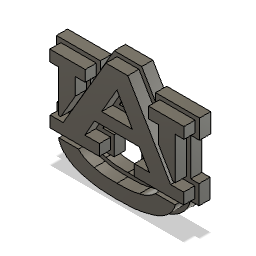
AU_void v3 (Autodesk Fusion 360 design; units mm, degrees)
Autodesk Fusion 360 part; units mm, degrees
sketch "Sketch1" plane through (0, 0, 0) normal (0, 0, 1) x (1, 0, 0)
  line L0 (-1.6004, 6.7897) -> (1.524, 6.7897)
  line L1 (1.524, 6.7897) -> (3.1002, 4.0732)
  line L2 (8.1251, 4.9997) -> (3.1021, 4.9997)
  line L3 (3.1021, 4.9997) -> (3.1002, 4.0732)
  line L4 (8.1251, 4.9997) -> (8.1251, 2.794)
  line L5 (8.1251, 2.794) -> (7.112, 2.794)
  line L6 (7.112, 2.794) -> (7.112, -1.524)
  line L7 (7.112, -1.524) -> (8.0633, -1.524)
  line L8 (8.0633, -1.524) -> (8.0633, -3.7222)
  line L9 (8.0633, -3.7222) -> (7.0698, -3.7222)
  line L10 (3.5709, 4.5364) -> (7.6215, 4.5364)
  line L11 (7.6215, 4.5364) -> (7.6215, 3.2693)
  line L12 (7.6215, 3.2693) -> (6.6294, 3.2693)
  line L13 (6.6294, 3.2693) -> (6.6294, -1.524)
  line L14 (6.6294, -1.524) -> (6.3679, -1.524)
  line L15 (6.3679, -1.524) -> (4.6978, 1.3381)
  line L16 (4.6978, 1.3381) -> (4.6978, 3.2693)
  line L17 (4.6978, 3.2693) -> (3.5709, 3.2693)
  line L18 (3.5709, 3.2693) -> (3.5709, 4.5364)
  line L19 (7.112, 2.794) -> (3.81, 2.794) construction
  line L20 (4.2503, 2.794) -> (4.2503, 2.032) construction
  line L21 (4.0893, 2.3382) -> (3.6031, 3.1299) construction
  line L22 (3.81, 2.794) -> (4.2503, 2.077) construction
  line L23 (4.2503, 2.794) -> (4.2503, 2.077)
  line L24 (3.81, 2.794) -> (4.2503, 2.077)
  line L25 (4.2503, 2.794) -> (4.2503, 2.077)
  line L26 (4.2503, 2.794) -> (3.81, 2.794)
  line L27 (3.81, 2.794) -> (-8.1806, 2.794) construction
  line L28 (-1.7889, 1.3156) -> (1.3724, 6.7897) construction
  line L29 (-1.7889, 1.3156) -> (1.722, 1.3156) construction
  line L30 (-0.0473, 4.3314) -> (1.722, 1.3156) construction
  line L31 (-0.0473, 4.3314) -> (-1.7889, 1.3156)
  line L32 (1.722, 1.3156) -> (-1.7889, 1.3156)
  line L33 (-0.0473, 4.3314) -> (1.722, 1.3156)
  line L34 (-0.0444, 3.4835) -> (0.9772, 1.7422)
  line L35 (-1.05, 1.7422) -> (0.9772, 1.7422)
  line L36 (-1.05, 1.7422) -> (-0.0444, 3.4835)
  line L37 (-0.2083, 6.3583) -> (1.397, 6.3583) construction
  line L38 (6.0908, -1.9713) -> (7.5853, -1.9713) construction
  line L39 (7.5853, -1.9713) -> (7.5853, -3.2478) construction
  line L40 (7.5853, -3.2478) -> (1.9477, -3.2478) construction
  line L41 (1.9477, -3.2478) -> (1.9477, -1.9713) construction
  line L42 (1.9477, -1.9713) -> (6.0908, -1.9713) construction
  line L43 (1.9477, -1.9713) -> (7.5853, -1.9713) construction
  line L44 (7.5853, -1.9713) -> (7.5853, -3.2478) construction
  line L45 (7.5853, -3.2478) -> (1.9477, -3.2478) construction
  line L46 (1.9477, -3.2478) -> (1.9477, -1.9713) construction
  line L47 (1.9477, -1.9713) -> (7.5853, -1.9713)
  line L48 (7.5853, -1.9713) -> (7.5853, -3.2478)
  line L49 (7.5853, -3.2478) -> (1.9477, -3.2478)
  line L50 (1.9477, -3.2478) -> (1.9477, -1.9713)
  line L51 (6.0908, -1.9713) -> (1.1131, 6.5067) construction
  line L52 (-0.0473, 4.3314) -> (-0.0473, 7.112) construction
  line L53 (-0.0473, 6.3583) -> (1.2002, 6.3583)
  line L54 (1.2002, 6.3583) -> (6.0908, -1.9713)
  line L55 (7.0698, -3.7222) -> (1.524, -3.7222) construction
  line L56 (1.524, -3.7222) -> (8.0633, -3.7222)
  line L57 (8.0633, -3.7222) -> (8.0633, -1.524)
  line L58 (8.0633, -1.524) -> (1.524, -1.524)
  line L59 (1.524, -1.524) -> (1.524, -3.7222)
  line L60 (2.8589, -1.524) -> (2.2352, -0.4826)
  line L61 (2.2352, -0.4826) -> (-2.3352, -0.4826) construction
  line L62 (-2.3352, -0.4826) -> (-2.9184, -1.5115) construction
  line L63 (-2.9184, -1.5115) -> (-2.3352, -0.4826)
  line L64 (-2.3352, -0.4826) -> (2.2352, -0.4826)
  line L65 (1.9477, -1.9713) -> (-3.9726, -1.9713) construction
  line L66 (3.2581, -1.2849) -> (2.4989, -0.0173)
  line L67 (-2.6063, -0.0173) -> (2.4989, -0.0173)
  line L68 (-3.717, -1.9768) -> (-2.6063, -0.0173)
  line L69 (-1.6175, -1.9768) -> (-3.717, -1.9768)
  line L70 (-0.0473, 7.112) -> (-0.0473, -8.382)
  line L71 (-0.0473, 6.3583) -> (-1.2948, 6.3583)
  line L72 (-1.2948, 6.3583) -> (-6.1854, -1.9713)
  line L73 (-4.345, 2.794) -> (-3.9046, 2.794)
  line L74 (-3.9046, 2.794) -> (-4.345, 2.077) construction
  line L75 (-4.345, 2.794) -> (-4.345, 2.032) construction
  line L76 (-4.7924, 1.3381) -> (-4.7924, 3.2693)
  line L77 (-4.7924, 3.2693) -> (-3.6655, 3.2693)
  line L78 (-3.6655, 3.2693) -> (-3.6655, 4.5364)
  line L79 (-3.6655, 4.5364) -> (-7.7162, 4.5364)
  line L80 (-7.7162, 4.5364) -> (-7.7162, 3.2693)
  line L81 (-7.7162, 3.2693) -> (-6.724, 3.2693)
  line L82 (-6.724, 3.2693) -> (-6.724, -1.524)
  line L83 (-6.4625, -1.524) -> (-4.7924, 1.3381)
  line L84 (-2.0423, -3.2478) -> (-2.0423, -1.9713)
  line L85 (-7.68, -3.2478) -> (-2.0423, -3.2478)
  line L86 (-2.0423, -1.9713) -> (-7.68, -1.9713)
  line L87 (-7.68, -1.9713) -> (-7.68, -3.2478)
  line L88 (-8.2198, 4.9997) -> (-3.1968, 4.9997)
  line L89 (-3.1968, 4.9997) -> (-3.1948, 4.0732)
  line L90 (-1.6186, 6.7897) -> (-3.1948, 4.0732)
  line L91 (-8.2198, 4.9997) -> (-8.2198, 2.794)
  line L92 (-8.2198, 2.794) -> (-7.2066, 2.794)
  line L93 (-7.2066, 2.794) -> (-7.2066, -1.524)
  line L94 (-8.158, -1.524) -> (-1.6186, -1.524)
  line L95 (-8.158, -3.7222) -> (-8.158, -1.524)
  line L96 (-1.6186, -3.7222) -> (-8.158, -3.7222)
  line L97 (-1.6186, -1.524) -> (-1.6186, -3.7222)
  line L98 (-3.9046, 2.794) -> (-4.345, 2.077)
  line L99 (-4.345, 2.794) -> (-4.345, 2.077)
  spline S0 degree 5 poles (6.586, -3.7222) (6.5894, -3.728) (6.595, -3.7414) (6.5992, -3.7671) (6.5964, -3.8127) (6.5791, -3.8881) (6.5484, -3.9806) (6.5051, -4.0876) (6.4506, -4.2047) (6.3866, -4.3267) (6.315, -4.4484) (6.2377, -4.5654) (6.1562, -4.6747) (6.0718, -4.7756) (5.9853, -4.8687) (5.8972, -4.9557) (5.8075, -5.0384) (5.7161, -5.1186) (5.6223, -5.197) (5.5253, -5.2738) (5.4244, -5.3488) (5.3189, -5.4218) (5.2086, -5.492) (5.0937, -5.5593) (4.9747, -5.6232) (4.8522, -5.6836) (4.7269, -5.7404) (4.5992, -5.7939) (4.469, -5.8442) (4.3363, -5.8918) (4.2007, -5.937) (4.0623, -5.9803) (3.9209, -6.0219) (3.7773, -6.062) (3.6323, -6.1004) (3.4869, -6.137) (3.3424, -6.1715) (3.1999, -6.2038) (3.0603, -6.2335) (2.9241, -6.2606) (2.7918, -6.2849) (2.6891, -6.3022) (2.6138, -6.3139) (2.5645, -6.3211) (2.54, -6.3246) knots 0 0 0 0 0 0 0.025 0.05 0.075 0.1 0.125 0.15 0.175 0.2 0.225 0.25 0.275 0.3 0.325 0.35 0.375 0.4 0.425 0.45 0.475 0.5 0.525 0.55 0.575 0.6 0.625 0.65 0.675 0.7 0.725 0.75 0.775 0.8 0.825 0.85 0.875 0.9 0.925 0.95 0.975 1 1 1 1 1 1
  spline S1 degree 5 poles (2.54, -6.3246) (2.5106, -6.3304) (2.4526, -6.3417) (2.3675, -6.3575) (2.258, -6.3763) (2.1277, -6.3959) (2.0038, -6.4118) (1.8859, -6.4241) (1.7731, -6.4331) (1.6641, -6.4395) (1.5572, -6.4441) (1.4506, -6.4476) (1.3424, -6.4509) (1.2312, -6.4544) (1.1162, -6.4587) (0.997, -6.4637) (0.8738, -6.4693) (0.7474, -6.4753) (0.6189, -6.4814) (0.49, -6.4873) (0.3629, -6.4928) (0.2397, -6.4975) (0.1224, -6.5014) (0.0127, -6.5041) (-0.088, -6.5056) (-0.1793, -6.5059) (-0.2446, -6.5052) (-0.2891, -6.504) (-0.3168, -6.503) (-0.3302, -6.5024) knots 0 0 0 0 0 0 0.04 0.08 0.12 0.16 0.2 0.24 0.28 0.32 0.36 0.4 0.44 0.48 0.52 0.56 0.6 0.64 0.68 0.72 0.76 0.8 0.84 0.88 0.92 0.96 1 1 1 1 1 1
  spline S2 degree 5 poles (4.3524, -3.7222) (4.3464, -3.7267) (4.3343, -3.7362) (4.3151, -3.7517) (4.2876, -3.7748) (4.25, -3.8077) (4.2089, -3.8446) (4.1638, -3.8854) (4.1141, -3.9296) (4.0591, -3.9768) (3.998, -4.0261) (3.9304, -4.0769) (3.8564, -4.1283) (3.7771, -4.1794) (3.6938, -4.2293) (3.6084, -4.2772) (3.5226, -4.3225) (3.4376, -4.3647) (3.354, -4.4036) (3.2714, -4.4393) (3.1891, -4.4722) (3.1058, -4.5025) (3.0205, -4.5307) (2.9322, -4.5571) (2.8403, -4.582) (2.7446, -4.6055) (2.6648, -4.6232) (2.6031, -4.6359) (2.5612, -4.6442) (2.54, -4.6482) knots 0 0 0 0 0 0 0.04 0.08 0.12 0.16 0.2 0.24 0.28 0.32 0.36 0.4 0.44 0.48 0.52 0.56 0.6 0.64 0.68 0.72 0.76 0.8 0.84 0.88 0.92 0.96 1 1 1 1 1 1
  spline S3 degree 5 poles (2.54, -4.6482) (2.5205, -4.6529) (2.4818, -4.6621) (2.4248, -4.6757) (2.3508, -4.6933) (2.2614, -4.7145) (2.175, -4.7347) (2.0909, -4.7539) (2.0081, -4.772) (1.925, -4.7891) (1.8398, -4.8049) (1.7508, -4.8194) (1.6565, -4.8326) (1.5561, -4.8444) (1.4493, -4.855) (1.3367, -4.8643) (1.2188, -4.8725) (1.097, -4.8797) (0.9725, -4.8859) (0.8469, -4.8913) (0.7217, -4.8958) (0.5984, -4.8996) (0.4784, -4.9025) (0.3627, -4.9046) (0.2519, -4.9059) (0.1463, -4.9065) (0.0661, -4.9064) (0.0085, -4.9059) (-0.0289, -4.9055) (-0.0473, -4.9052) knots 0 0 0 0 0 0 0.04 0.08 0.12 0.16 0.2 0.24 0.28 0.32 0.36 0.4 0.44 0.48 0.52 0.56 0.6 0.64 0.68 0.72 0.76 0.8 0.84 0.88 0.92 0.96 1 1 1 1 1 1
  spline S4 degree 3 poles (2.452, -4.2392) (2.4488, -4.24) (2.4457, -4.2407) (2.4426, -4.2415) (1.9896, -4.35) (1.7292, -4.4202) (1.1911, -4.4549) (0.7682, -4.4821) (0.2826, -4.4916) (-0.0414, -4.487) knots -0.003853 -0.003853 -0.003853 -0.003853 0 0 0 0.559939 0.559939 0.559939 1 1 1 1
  spline S5 degree 3 poles (2.6128, -6.751) (2.1368, -6.8452) (1.7587, -6.8706) (1.4212, -6.8811) (1.1206, -6.8905) (0.7741, -6.9083) (0.4206, -6.9231) (0.1093, -6.9362) (-0.1594, -6.9426) (-0.3488, -6.9345) knots 0.003026 0.003026 0.003026 0.003026 0.375759 0.375759 0.375759 0.707718 0.707718 0.707718 1 1 1 1
  spline S6 degree 3 poles (7.0353, -3.7222) (7.0414, -3.7958) (7.0259, -3.8546) (7.0166, -3.9058) (6.977, -4.1227) (6.8834, -4.3231) (6.753, -4.5541) (6.5674, -4.8828) (6.3122, -5.1669) (6.0785, -5.3753) (5.7717, -5.6489) (5.3994, -5.9085) (4.9752, -6.1021) (4.4374, -6.3475) (3.8359, -6.5079) (3.2646, -6.6318) (3.0354, -6.6816) (2.8173, -6.7216) (2.6128, -6.751) knots 0.024795 0.024795 0.024795 0.024795 0.054071 0.054071 0.054071 0.178055 0.178055 0.178055 0.354527 0.354527 0.354527 0.586219 0.586219 0.586219 0.879934 0.879934 0.879934 0.997732 0.997732 0.997732 0.997732
  spline S7 degree 3 poles (3.7035, -3.7222) (3.6472, -3.7643) (3.5846, -3.807) (3.5132, -3.8495) (3.3139, -3.9684) (3.1123, -4.0616) (2.9062, -4.1275) (2.7773, -4.1687) (2.6302, -4.2052) (2.4615, -4.2374) (2.4583, -4.238) (2.4551, -4.2386) (2.452, -4.2392) knots 0.345635 0.345635 0.345635 0.345635 0.463712 0.463712 0.463712 0.793602 0.793602 0.793602 1 1 1 1.003585 1.003585 1.003585 1.003585
  spline S8 degree 5 poles (-4.447, -3.7222) (-4.4411, -3.7267) (-4.4289, -3.7362) (-4.4098, -3.7517) (-4.3823, -3.7748) (-4.3446, -3.8077) (-4.3035, -3.8446) (-4.2584, -3.8854) (-4.2088, -3.9296) (-4.1538, -3.9768) (-4.0926, -4.0261) (-4.025, -4.0769) (-3.9511, -4.1283) (-3.8717, -4.1794) (-3.7884, -4.2293) (-3.703, -4.2772) (-3.6172, -4.3225) (-3.5322, -4.3647) (-3.4486, -4.4036) (-3.366, -4.4393) (-3.2837, -4.4722) (-3.2004, -4.5025) (-3.1151, -4.5307) (-3.0268, -4.5571) (-2.935, -4.582) (-2.8392, -4.6055) (-2.7594, -4.6232) (-2.6977, -4.6359) (-2.6558, -4.6442) (-2.6346, -4.6482) knots 0 0 0 0 0 0 0.04 0.08 0.12 0.16 0.2 0.24 0.28 0.32 0.36 0.4 0.44 0.48 0.52 0.56 0.6 0.64 0.68 0.72 0.76 0.8 0.84 0.88 0.92 0.96 1 1 1 1 1 1
  line L100 (4.488, -3.618) -> (4.2167, -3.8265)
  line L101 (2.7796, -4.6024) -> (2.3004, -4.694)
  line L102 (-4.5826, -3.618) -> (-4.3114, -3.8265)
  line L103 (-2.8742, -4.6024) -> (-2.395, -4.694)
  spline S9 degree 5 poles (-2.6346, -4.6482) (-2.6151, -4.6529) (-2.5765, -4.6621) (-2.5195, -4.6757) (-2.4454, -4.6933) (-2.3561, -4.7145) (-2.2697, -4.7347) (-2.1856, -4.7539) (-2.1028, -4.772) (-2.0197, -4.7891) (-1.9345, -4.8049) (-1.8455, -4.8194) (-1.7512, -4.8326) (-1.6507, -4.8444) (-1.544, -4.855) (-1.4313, -4.8643) (-1.3134, -4.8725) (-1.1916, -4.8797) (-1.0671, -4.8859) (-0.9415, -4.8913) (-0.8163, -4.8958) (-0.6931, -4.8996) (-0.5731, -4.9025) (-0.4573, -4.9046) (-0.3465, -4.9059) (-0.2409, -4.9065) (-0.1608, -4.9064) (-0.1031, -4.9059) (-0.0657, -4.9055) (-0.0473, -4.9052) knots 0 0 0 0 0 0 0.04 0.08 0.12 0.16 0.2 0.24 0.28 0.32 0.36 0.4 0.44 0.48 0.52 0.56 0.6 0.64 0.68 0.72 0.76 0.8 0.84 0.88 0.92 0.96 1 1 1 1 1 1
  line L104 (2.822, -4.5806) -> (2.258, -4.7158)
  line L105 (0.1863, -4.9085) -> (-0.281, -4.9019)
  line L106 (-2.9167, -4.5806) -> (-2.3526, -4.7158)
  line L107 (-0.281, -4.9085) -> (0.1863, -4.9019)
  spline S10 degree 3 poles (-2.5466, -4.2392) (-2.5435, -4.24) (-2.5403, -4.2407) (-2.5372, -4.2415) (-2.0842, -4.35) (-1.8238, -4.4202) (-1.2858, -4.4549) (-0.8629, -4.4821) (-0.3772, -4.4916) (-0.0532, -4.487) knots -0.003853 -0.003853 -0.003853 -0.003853 0 0 0 0.559939 0.559939 0.559939 1 1 1 1
  spline S11 degree 3 poles (-3.7982, -3.7222) (-3.7418, -3.7643) (-3.6792, -3.807) (-3.6078, -3.8495) (-3.4085, -3.9684) (-3.2069, -4.0616) (-3.0008, -4.1275) (-2.8719, -4.1687) (-2.7249, -4.2052) (-2.5561, -4.2374) (-2.5529, -4.238) (-2.5498, -4.2386) (-2.5466, -4.2392) knots 0.345635 0.345635 0.345635 0.345635 0.463712 0.463712 0.463712 0.793602 0.793602 0.793602 1 1 1 1.003585 1.003585 1.003585 1.003585
  spline S12 degree 5 poles (-6.6806, -3.7222) (-6.6841, -3.728) (-6.6896, -3.7414) (-6.6938, -3.7671) (-6.6911, -3.8127) (-6.6738, -3.8881) (-6.6431, -3.9806) (-6.5998, -4.0876) (-6.5452, -4.2047) (-6.4813, -4.3267) (-6.4097, -4.4484) (-6.3323, -4.5654) (-6.2509, -4.6747) (-6.1665, -4.7756) (-6.08, -4.8687) (-5.9918, -4.9557) (-5.9022, -5.0384) (-5.8107, -5.1186) (-5.7169, -5.197) (-5.6199, -5.2738) (-5.519, -5.3488) (-5.4135, -5.4218) (-5.3032, -5.492) (-5.1883, -5.5593) (-5.0693, -5.6232) (-4.9469, -5.6836) (-4.8216, -5.7404) (-4.6938, -5.7939) (-4.5636, -5.8442) (-4.4309, -5.8918) (-4.2954, -5.937) (-4.1569, -5.9803) (-4.0156, -6.0219) (-3.872, -6.062) (-3.7269, -6.1004) (-3.5816, -6.137) (-3.4371, -6.1715) (-3.2946, -6.2038) (-3.155, -6.2335) (-3.0188, -6.2606) (-2.8864, -6.2849) (-2.7837, -6.3022) (-2.7085, -6.3139) (-2.6591, -6.3211) (-2.6346, -6.3246) knots 0 0 0 0 0 0 0.025 0.05 0.075 0.1 0.125 0.15 0.175 0.2 0.225 0.25 0.275 0.3 0.325 0.35 0.375 0.4 0.425 0.45 0.475 0.5 0.525 0.55 0.575 0.6 0.625 0.65 0.675 0.7 0.725 0.75 0.775 0.8 0.825 0.85 0.875 0.9 0.925 0.95 0.975 1 1 1 1 1 1
  line L108 (5.407, -3.8375) -> (7.7649, -3.6069)
  line L109 (3.0533, -6.2522) -> (2.0267, -6.397)
  line L110 (-5.5016, -3.8375) -> (-7.8596, -3.6069)
  line L111 (-3.1479, -6.2522) -> (-2.1214, -6.397)
  spline S13 degree 5 poles (-2.6346, -6.3246) (-2.6053, -6.3304) (-2.5472, -6.3417) (-2.4622, -6.3575) (-2.3527, -6.3763) (-2.2224, -6.3959) (-2.0985, -6.4118) (-1.9806, -6.4241) (-1.8678, -6.4331) (-1.7588, -6.4395) (-1.6519, -6.4441) (-1.5452, -6.4476) (-1.437, -6.4509) (-1.3259, -6.4544) (-1.2109, -6.4587) (-1.0916, -6.4637) (-0.9685, -6.4693) (-0.842, -6.4753) (-0.7135, -6.4814) (-0.5847, -6.4873) (-0.4576, -6.4928) (-0.3343, -6.4975) (-0.217, -6.5014) (-0.1074, -6.5041) (-0.0066, -6.5056) (0.0847, -6.5059) (0.1499, -6.5052) (0.1944, -6.504) (0.2222, -6.503) (0.2356, -6.5024) knots 0 0 0 0 0 0 0.04 0.08 0.12 0.16 0.2 0.24 0.28 0.32 0.36 0.4 0.44 0.48 0.52 0.56 0.6 0.64 0.68 0.72 0.76 0.8 0.84 0.88 0.92 0.96 1 1 1 1 1 1
  line L112 (2.8691, -6.2591) -> (2.2109, -6.3901)
  line L113 (-0.109, -6.5119) -> (-0.5514, -6.4929)
  line L114 (-2.9638, -6.2591) -> (-2.3055, -6.3901)
  line L115 (0.0143, -6.5119) -> (0.4568, -6.4929)
  spline S14 degree 3 poles (-2.7075, -6.751) (-2.2315, -6.8452) (-1.8534, -6.8706) (-1.5158, -6.8811) (-1.2152, -6.8905) (-0.8687, -6.9083) (-0.5152, -6.9231) (-0.204, -6.9362) (0.0647, -6.9426) (0.2542, -6.9345) knots 0.003026 0.003026 0.003026 0.003026 0.375759 0.375759 0.375759 0.707718 0.707718 0.707718 1 1 1 1
  spline S15 degree 3 poles (-7.13, -3.7222) (-7.1361, -3.7958) (-7.1205, -3.8546) (-7.1112, -3.9058) (-7.0717, -4.1227) (-6.978, -4.3231) (-6.8476, -4.5541) (-6.662, -4.8828) (-6.4068, -5.1669) (-6.1731, -5.3753) (-5.8663, -5.6489) (-5.494, -5.9085) (-5.0698, -6.1021) (-4.532, -6.3475) (-3.9305, -6.5079) (-3.3592, -6.6318) (-3.1301, -6.6816) (-2.912, -6.7216) (-2.7075, -6.751) knots 0.024795 0.024795 0.024795 0.024795 0.054071 0.054071 0.054071 0.178055 0.178055 0.178055 0.354527 0.354527 0.354527 0.586219 0.586219 0.586219 0.879934 0.879934 0.879934 0.997732 0.997732 0.997732 0.997732
  line L116 (-2.9184, -1.5115) -> (-2.3352, -0.4826)
  line L117 (2.2352, -0.4826) -> (2.8589, -1.524)
  line L118 (1.524, -1.524) -> (1.524, -3.7222)
  line L119 (3.0088, -0.8687) -> (3.6712, -1.9748)
  line L120 (3.0088, -0.8687) -> (4.298, -0.8687) construction
  line L121 (3.6712, -1.9748) -> (1.9477, -1.9713)
  line L122 (-2.839, -1.3714) -> (-2.9255, -1.524)
  line L123 (-2.839, -1.3714) -> (-2.6635, -1.3714) construction
  line L124 (4.3524, -3.7222) -> (3.7035, -3.7222)
  line L125 (-0.0532, -4.487) -> (-0.0414, -4.487)
  line L126 (-1.6004, 6.7897) -> (-1.6186, 6.7897)
  point P0 (6.5532, -3.9624)
  point P1 (6.2484, -4.5466)
  point P2 (5.8166, -5.0292)
  point P3 (5.334, -5.4102)
  point P4 (4.7244, -5.7404)
  point P5 (4.0132, -5.9944)
  point P6 (3.2258, -6.1976)
  point P7 (1.8542, -6.4262)
  point P8 (1.3208, -6.4516)
  point P9 (0.7112, -6.477)
  point P10 (0.0762, -6.5024)
  point P11 (4.191, -3.8608)
  point P12 (3.9116, -4.0894)
  point P13 (3.4798, -4.3434)
  point P14 (3.048, -4.5212)
  point P15 (2.1082, -4.7498)
  point P16 (1.7018, -4.826)
  point P17 (1.143, -4.8768)
  point P18 (0.4826, -4.9022)
  point P19 (-4.2856, -3.8608)
  point P20 (-4.0062, -4.0894)
  point P21 (-3.5744, -4.3434)
  point P22 (-3.1426, -4.5212)
  point P23 (-2.2028, -4.7498)
  point P24 (-1.7964, -4.826)
  point P25 (-1.2376, -4.8768)
  point P26 (-0.5772, -4.9022)
  point P27 (-6.6478, -3.9624)
  point P28 (-6.343, -4.5466)
  point P29 (-5.9112, -5.0292)
  point P30 (-5.4286, -5.4102)
  point P31 (-4.819, -5.7404)
  point P32 (-4.1078, -5.9944)
  point P33 (-3.3204, -6.1976)
  point P34 (-1.9488, -6.4262)
  point P35 (-1.4154, -6.4516)
  point P36 (-0.8058, -6.477)
  point P37 (-0.1708, -6.5024)
  dimension "d1" = 0.4266
  dimension "d5" = 59.083
  dimension "d6" = 119.545
  constraint horizontal L0
  constraint horizontal L2
  constraint perpendicular L2 L4
  constraint perpendicular L4 L5
  constraint perpendicular L5 L6
  constraint perpendicular L6 L7
  constraint perpendicular L7 L8
  constraint perpendicular L8 L9
  constraint perpendicular L10 L11
  constraint perpendicular L11 L12
  constraint perpendicular L12 L13
  constraint perpendicular L11 L14
  constraint perpendicular L12 L16
  constraint perpendicular L16 L17
  constraint perpendicular L10 L18
  constraint perpendicular L16 L19
  constraint coincident L19 L20.start
  constraint perpendicular L19 L20
  constraint coincident L20 L22.end
  constraint parallel L21 L22
  constraint parallel L22 L24
  constraint parallel L26 L27
  constraint coincident L0 L28.end
  constraint parallel L0 L29
  constraint coincident L28 L30.start
  constraint parallel L29 L32
  constraint parallel L30 L33
  constraint horizontal L37
  constraint parallel L27 L38
  constraint perpendicular L38 L39
  constraint perpendicular L39 L40
  constraint perpendicular L40 L41
  constraint perpendicular L41 L42
  constraint horizontal L43
  constraint vertical L44
  constraint horizontal L45
  constraint vertical L46
  constraint horizontal L47
  constraint vertical L48
  constraint horizontal L49
  constraint vertical L50
  constraint perpendicular L0 L52
  constraint coincident L52 L53.start
  constraint coincident L37 L53.start
  constraint coincident L37 L53.end
  constraint coincident L51 L53.end
  constraint perpendicular L39 L55
  constraint horizontal L56
  constraint vertical L57
  constraint horizontal L58
  constraint vertical L59
  constraint coincident L58 L60.start
  constraint parallel L58 L61
  constraint parallel L62 L63
  constraint parallel L61 L64
  constraint perpendicular L59 L65
  constraint perpendicular L65 L70
  constraint symmetric L0.end L70 L90.start
  constraint symmetric L1.end L70 L89.end
  constraint symmetric L2.start L70 L88.start
  constraint symmetric L2.end L70 L88.end
  constraint symmetric L4.end L70 L91.end
  constraint symmetric L5.end L70 L92.end
  constraint symmetric L6.end L70 L93.end
  constraint symmetric L7.end L70 L94.start
  constraint symmetric L10.end L70 L79.end
  constraint symmetric L11.end L70 L80.end
  constraint symmetric L12.end L70 L81.end
  constraint symmetric L13.end L70 L82.end
  constraint symmetric L14.end L70 L83.start
  constraint symmetric L15.end L70 L76.start
  constraint symmetric L16.end L70 L76.end
  constraint symmetric L17.end L70 L77.end
  constraint symmetric L10.start L70 L78.end
  constraint symmetric L19.end L70 L73.end
  constraint symmetric L20.start L70 L73.start
  constraint symmetric L20.end L70 L75.end
  constraint symmetric L22.end L70 L74.end
  constraint symmetric L38.start L70 L72.end
  constraint symmetric L39.end L70 L85.start
  constraint symmetric L41.end L70 L84.end
  constraint symmetric L38.end L70 L86.end
  constraint symmetric L40.end L70 L84.start
  constraint symmetric L53.start L70 L71.start
  constraint symmetric L53.end L70 L71.end
  constraint symmetric L55.end L70 L96.start
  constraint symmetric L8.end L70 L95.start
  constraint symmetric L58.end L70 L94.end
  constraint parallel L74 L98
  constraint coincident L56 S0.start
  constraint coincident L55 S0.start
  constraint coincident L56 S2.start
  constraint coincident L70 S3.end
  constraint coincident L55 S6.start
  constraint coincident L55 S7.start
  constraint midpoint S2.start L100
  constraint midpoint S2.end L101
  constraint midpoint S2.end L104
  constraint midpoint S3.end L105
  constraint midpoint S0.start L108
  constraint midpoint S0.end L109
  constraint midpoint S0.end L112
  constraint midpoint S1.end L113
  constraint symmetric L70 S0.start S12.start
  constraint symmetric L70 P0 P27
  constraint symmetric L70 P1 P28
  constraint symmetric L70 P2 P29
  constraint symmetric L70 P3 P30
  constraint symmetric L70 P4 P31
  constraint symmetric L70 P5 P32
  constraint symmetric L70 P6 P33
  constraint symmetric L70 S0.end S12.end
  constraint symmetric L70 P7 P34
  constraint symmetric L70 P8 P35
  constraint symmetric L70 P9 P36
  constraint symmetric L70 P10 P37
  constraint symmetric L70 S1.end S13.end
  constraint symmetric L70 S2.start S8.start
  constraint symmetric L70 P11 P19
  constraint symmetric L70 P12 P20
  constraint symmetric L70 P13 P21
  constraint symmetric L70 P14 P22
  constraint symmetric L70 S2.end S8.end
  constraint symmetric L70 P15 P23
  constraint symmetric L70 P16 P24
  constraint symmetric L70 P17 P25
  constraint symmetric L70 P18 P26
  constraint symmetric L70 S3.end S9.end
  constraint symmetric L70 S4.start S10.start
  constraint symmetric L70 S4.end S10.end
  constraint symmetric L70 S4 S10
  constraint symmetric L70 S5.start S14.start
  constraint symmetric L70 S5.end S14.end
  constraint symmetric L70 S5 S14
  constraint symmetric L70 S6.start S15.start
  constraint symmetric L70 S6 S15
  constraint symmetric L70 S7.start S11.start
  constraint symmetric L70 S7 S11
  constraint symmetric L70 L100.start L102.start
  constraint symmetric L70 L100.end L102.end
  constraint symmetric L70 L101.start L103.start
  constraint symmetric L70 L101.end L103.end
  constraint symmetric L70 L104.start L106.start
  constraint symmetric L70 L104.end L106.end
  constraint symmetric L70 L105.start L107.start
  constraint symmetric L70 L105.end L107.end
  constraint symmetric L70 L108.start L110.start
  constraint symmetric L70 L108.end L110.end
  constraint symmetric L70 L109.start L111.start
  constraint symmetric L70 L109.end L111.end
  constraint symmetric L70 L112.start L114.start
  constraint symmetric L70 L112.end L114.end
  constraint symmetric L70 L113.start L115.start
  constraint symmetric L70 L113.end L115.end
  constraint parallel L63 L116
  constraint parallel L60 L117
  constraint horizontal L120
  constraint coincident L66 L119.start
  constraint parallel L60 L66
  constraint parallel L64 L67
  constraint parallel L63 L68
  constraint horizontal L123
  constraint coincident L116 L122.start
  constraint coincident L94 L122.end
  constraint parallel L55 L124
  constraint perpendicular L70 L125
  constraint parallel L0 L126
  measures "d5" angle of L119 L120
  measures "d6" angle of L122 L123
extrude "Extrude1" add sketch "Sketch1" along normal blind 2.54 contours L32 L33 L53 L54 L58 L66 L67 L70 L119 | L31 L32 L67 L68 L70 L71 L72 L94 | L47 L54 L58 L119 | L68 L72 L86 L94 | L47 L48 L49 L50 L119 L121 | L10 L11 L12 L13 L14 L15 L16 L17 L18 L58 | L68 L69 L84 L85 L86 L87 | L76 L77 L78 L79 L80 L81 L82 L83 L94 | L56 L70 S0 S1 S2 S3 L104 | L70 L96 S8 S9 L106 S12 S13 makes body 1 at (6.6294, 1.6715, 0.8467) makes body 2 at (-6.724, 1.6715, 0.8467) makes body 3 at (0.6555, -5.951, 0) makes body 4 at (-3.0022, 2.05, 0)
extrude "Extrude4" add sketch "Sketch1" along normal blind 1.27 contours L0 L70 L71 L72 L76 L77 L78 L79 L80 L81 L82 L83 L88 L89 L90 L91 L92 L93 L94 L126 | L0 L1 L2 L3 L4 L5 L6 L10 L11 L12 L13 L15 L16 L17 L18 L53 L54 L58 L70 | L31 L32 L35 L36 L70 | L32 L33 L34 L35 L36 L70 | L7 L8 L9 L14 L47 L48 L49 L50 L54 L56 L57 L58 L59 L118 L119 L124 | L69 L72 L84 L85 L86 L87 L94 L95 L96 L97 | L58 L60 L64 L66 L67 L70 L117 L119 | L68 L69 L84 L86 L94 L97 | L63 L64 L67 L68 L70 L94 L116 L122 | L56 L70 S2 S3 S4 S7 L104 L124 L125 | L70 L96 S8 S9 L106 S10 S11 L125 | L56 L70 S0 S1 S5 S6 | L70 L96 S12 S13 S14 S15 bodies 2 3 1 4
ref_plane "WorkPlane1" through (-0.0473, 1.5553, 1.524) normal (0, 0, 1) x (1, 0, 0)
other "SpherePrimitive1"
scale "Scale1" factor 1 about (0, 0, 0) bodies 2
scale "Scale2" factor 3.5 about (0, 0, 0) bodies 2
extrude "Extrude2" [suppressed]
extrude "Extrude3" [suppressed]
